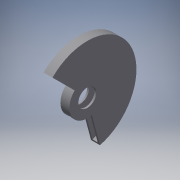
# Autodesk Inventor part: protector
Saved by Autodesk Inventor 2018 (Build 220112000, 112)
## iProperties
Created: 2021-07-10
Part Number: protector
Material: Genérico
Document SubType Name: Modeling
Designer: GABRIEL
Density: 1 g/cm^3
Appearance: Valor por defecto
Author: GABRIEL
Autodesk Inventor part; units mm, degrees
ref_plane "YZ Plane" through (0, 0, 0) normal (1, 0, 0) x (0, 1, 0)
ref_plane "XZ Plane" through (0, 0, 0) normal (0, 1, 0) x (-1, 0, 0)
ref_plane "XY Plane" through (0, 0, 0) normal (0, 0, 1) x (1, 0, 0)
sketch "Boceto1" plane through (0, 0, 0) normal (1, 0, 0) x (0, 1, 0)
  circle A0 centre (0, 0) radius 65
  line L0 (0, 0) -> (-45.9619, 45.9619)
  line L1 (0, 0) -> (65, 0) construction
  line L2 (0, 0) -> (16.8232, -62.7852)
  line L3 (0, 0) -> (65, 0) construction
  circle A1 centre (0, 0) radius 15
  dimension "d5" = 130
  dimension "d6" = 135
  dimension "d7" = 75
  dimension "d8" = 30
  constraints: 8 end point, 2 centre point, 2 coincident, 2 equal length, 2 horizontal, 2 point on circle
  measures "d5" diameter of A0
  measures "d6" angle of L1 L0
  measures "d7" angle of L2 L3
  measures "d8" diameter of A1
extrude "Extrusión1" add sketch "Boceto1" along normal blind 10 contours A0 L2 A1 L0 | A1 L2 L0 | L0 L2 A1 picked at (40.3579, 26.2595)
sketch "Boceto2" plane through (0, 3.8823, -14.4889) normal (0, -0.9659258, -0.258819) x (1, 0, 0)
  line L0 (2, -20) -> (8, -20)
  line L1 (8, -20) -> (8, -48)
  line L2 (8, -48) -> (2, -48)
  line L3 (2, -48) -> (2, -20)
  line L4 (10, 0) -> (10, 27.9904) projected
  line L5 (0, -50) -> (10, -50) projected
  point P0 (0, 15)
  dimension "d11" = 6
  dimension "d12" = 28
  dimension "d18" = 2
  constraints: 8 end point, 2 parallel, 1 horizontal, 1 perpendicular
  measures "d11" distance of L1.end L2.end
  measures "d12" distance of L0.end L1.end
  measures "d18" distance between parallel lines of L5 L2
revolve "Revolución1" cut sketch "Boceto2" angle 360 about axis through (2, 9.0587, -33.8074) along (1, 0, 0)
sketch "Boceto3" plane through (10, 0, 0) normal (1, 0, 0) x (0, 0, -1)
  circle A0 centre (0, 0) radius 10
  arc A1 (-10.6066, -10.6066) -> (14.4889, 3.8823) centre (0, 0) ccw projected
  dimension "d20" = 20
  constraints: 1 centre point, 1 concentric
  measures "d20" diameter of A0
extrude "Extrusión2" cut sketch "Boceto3" against normal blind 10
sketch "Boceto4" plane through (0, 0, 0) normal (-1, 0, 0) x (0, 0, 1)
  point P0 (0, 0)
sketch "Boceto5" plane through (0, 0, 0) normal (-1, 0, 0) x (0, 0, 1)
  arc A0 (46.9928, -0.8201) -> (0, 47) centre (0, 0) ccw
  circle A1 centre (16.5227, 44) radius 4
  circle A2 centre (33.5227, 32.9428) radius 4
  dimension "d23" = 47
  dimension "d24" = 8
  dimension "d25" = 8
  dimension "d28" = 17
  dimension "d29" = 44
  constraints: 4 point on circle, 3 centre point, 1 coincident
  measures "d23" radius of A0
  measures "d24" diameter of A1
  measures "d25" diameter of A2
  measures "d28" horizontal distance of A2.centre A1.centre
  measures "d29" vertical distance of point (0, 0) A1.centre
extrude "Extrusión3" cut sketch "Boceto5" against normal blind 2
